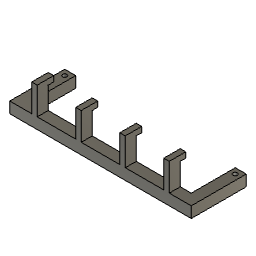
keys holder (Autodesk Fusion 360 design; units mm, degrees)
Autodesk Fusion 360 part; units mm, degrees
sketch "Sketch1" plane through (0, 0, 0) normal (0, 0, 1) x (1, 0, 0)
  line L0 (0, 0) -> (165, 0)
  line L1 (165, 0) -> (165, 50)
  line L2 (165, 50) -> (0, 50)
  line L3 (0, 50) -> (0, 0)
  line L4 (0, 50) -> (10, 50)
  line L5 (10, 50) -> (10, 0)
  line L6 (10, 0) -> (0, 0)
  line L7 (0, 0) -> (0, 50)
  line L8 (165, 50) -> (155, 50)
  line L9 (155, 50) -> (155, 0)
  line L10 (155, 0) -> (165, 0)
  line L11 (165, 0) -> (165, 50)
  line L12 (0, 10) -> (165, 10)
  line L13 (165, 10) -> (165, 0)
  line L14 (165, 0) -> (0, 0)
  line L15 (0, 0) -> (0, 10)
  dimension "d1" = 165
  dimension "d2" = 50
  dimension "d3" = 10
  dimension "d4" = 10
  dimension "d5" = 50
  constraint horizontal L0
  constraint vertical L1
  constraint horizontal L2
  constraint vertical L3
  constraint coincident L0.start L3.end
  constraint horizontal L4
  constraint vertical L5
  constraint horizontal L6
  constraint vertical L7
  constraint horizontal L8
  constraint vertical L9
  constraint horizontal L10
  constraint vertical L11
  constraint horizontal L12
  constraint vertical L13
  constraint horizontal L14
  constraint vertical L15
  constraint coincident L7 L12.start
  measures "d1" distance of L0.start L0.end
  measures "d2" distance of L0.start L2.end
  measures "d3" distance of L2.end L4.end
  measures "d4" distance of L1.end L8.end
  measures "d5" distance of L1.end L0.end
extrude "Extrude1" add sketch "Sketch1" along normal blind 10 contours L0 L3 L5 L6 L7 L12 L14 L15 | L0 L5 L9 L12 L14 | L2 L3 L4 L5 L7 L12 | L0 L1 L9 L10 L11 L12 L13 L14 | L1 L2 L8 L9 L11 L12
sketch "Sketch2" plane through (0, 0, 10) normal (0, 0, 1) x (-1, 0, 0)
  line L0 (-165, 0) -> (-165, -50)
  line L1 (-165, -50) -> (-155, -50)
  line L2 (-155, -50) -> (-155, -10)
  line L3 (-155, -10) -> (-10, -10)
  line L4 (-10, -10) -> (-10, -50)
  line L5 (-10, -50) -> (0, -50)
  line L6 (0, -50) -> (0, 0)
  line L7 (0, 0) -> (-165, 0)
  circle A0 centre (-5, -45) radius 2
  circle A1 centre (-160, -45) radius 2
  dimension "d8" = 4
  dimension "d9" = 4
  measures "d8" diameter of A0
  measures "d9" diameter of A1
extrude "Extrude2" cut sketch "Sketch2" against normal blind 10 contours A0 | A1
sketch "Sketch3" plane through (0, 0, 10) normal (0, 0, 1) x (-1, 0, 0)
  circle A0 centre (-160, -45) radius 2
  circle A1 centre (-5, -45) radius 2
  line L0 (-165, 0) -> (-165, -50)
  line L1 (-165, -50) -> (-155, -50)
  line L2 (-155, -50) -> (-155, -10)
  line L3 (-155, -10) -> (-10, -10)
  line L4 (-10, -10) -> (-10, -50)
  line L5 (-10, -50) -> (0, -50)
  line L6 (0, -50) -> (0, 0)
  line L7 (0, 0) -> (-165, 0)
  line L8 (0, 0) -> (-20, 0)
  line L9 (-20, 0) -> (-25, 0)
  line L10 (-25, 0) -> (-25, -10)
  line L11 (-25, -10) -> (-20, -10)
  line L12 (-20, -10) -> (-20, 0)
  line L13 (-25, 0) -> (-60, 0)
  line L14 (-60, 0) -> (-65, 0)
  line L15 (-65, 0) -> (-65, -10)
  line L16 (-65, -10) -> (-60, -10)
  line L17 (-60, -10) -> (-60, 0)
  line L18 (-65, 0) -> (-100, 0)
  line L19 (-100, 0) -> (-105, 0)
  line L20 (-105, 0) -> (-105, -10)
  line L21 (-105, -10) -> (-100, -10)
  line L22 (-100, -10) -> (-100, 0)
  line L23 (-105, 0) -> (-140, 0)
  line L24 (-140, 0) -> (-145, 0)
  line L25 (-145, 0) -> (-145, -10)
  line L26 (-145, -10) -> (-140, -10)
  line L27 (-140, -10) -> (-140, 0)
  dimension "d12" = 20
  dimension "d13" = 5
  dimension "d14" = 10
  dimension "d15" = 35
  dimension "d16" = 35
  dimension "d17" = 35
  constraint coincident L6.end L7.start
  constraint perpendicular L6 L8
  constraint horizontal L9
  constraint vertical L10
  constraint horizontal L11
  constraint vertical L12
  constraint perpendicular L10 L13
  constraint horizontal L14
  constraint vertical L15
  constraint horizontal L16
  constraint vertical L17
  constraint coincident L3 L15.end
  constraint perpendicular L15 L18
  constraint horizontal L19
  constraint vertical L20
  constraint horizontal L21
  constraint vertical L22
  constraint coincident L3 L20.end
  constraint perpendicular L20 L23
  constraint horizontal L24
  constraint vertical L25
  constraint horizontal L26
  constraint vertical L27
  constraint coincident L3 L25.end
  measures "d12" distance of L6.end L8.end
  measures "d13" distance of L8.end L9.end
  measures "d14" distance of L8.end L11.end
  measures "d15" distance of L9.end L13.end
  measures "d16" distance of L14.end L18.end
  measures "d17" distance of L19.end L23.end
extrude "Extrude3" add sketch "Sketch3" along normal blind 25 contours L3 L7 L24 L25 L26 L27 | L3 L7 L19 L20 L21 L22 | L3 L7 L14 L15 L16 L17 | L3 L7 L9 L10 L11 L12
sketch "Sketch4" plane through (0, 10, 0) normal (0, 1, 0) x (-1, 0, 0)
  line L0 (-155, 0) -> (-10, 0)
  line L1 (-10, 0) -> (-10, 10)
  line L2 (-10, 10) -> (-20, 10)
  line L3 (-20, 10) -> (-20, 35)
  line L4 (-20, 35) -> (-25, 35)
  line L5 (-25, 35) -> (-25, 10)
  line L6 (-25, 10) -> (-60, 10)
  line L7 (-60, 10) -> (-60, 35)
  line L8 (-60, 35) -> (-65, 35)
  line L9 (-65, 35) -> (-65, 10)
  line L10 (-65, 10) -> (-100, 10)
  line L11 (-100, 10) -> (-100, 35)
  line L12 (-100, 35) -> (-105, 35)
  line L13 (-105, 35) -> (-105, 10)
  line L14 (-105, 10) -> (-140, 10)
  line L15 (-140, 10) -> (-140, 35)
  line L16 (-140, 35) -> (-145, 35)
  line L17 (-145, 35) -> (-145, 10)
  line L18 (-145, 10) -> (-155, 10)
  line L19 (-155, 10) -> (-155, 0)
  line L20 (-20, 30) -> (-25, 30)
  line L21 (-25, 30) -> (-25, 35)
  line L22 (-25, 35) -> (-20, 35)
  line L23 (-20, 35) -> (-20, 30)
  line L24 (-60, 30) -> (-65, 30)
  line L25 (-65, 30) -> (-65, 35)
  line L26 (-65, 35) -> (-60, 35)
  line L27 (-60, 35) -> (-60, 30)
  line L28 (-100, 30) -> (-105, 30)
  line L29 (-105, 30) -> (-105, 35)
  line L30 (-105, 35) -> (-100, 35)
  line L31 (-100, 35) -> (-100, 30)
  line L32 (-140, 30) -> (-145, 30)
  line L33 (-145, 30) -> (-145, 35)
  line L34 (-145, 35) -> (-140, 35)
  line L35 (-140, 35) -> (-140, 30)
  constraint horizontal L20
  constraint vertical L21
  constraint horizontal L22
  constraint vertical L23
  constraint coincident L4.end L5.start
  constraint coincident L3 L20.start
  constraint horizontal L24
  constraint vertical L25
  constraint horizontal L26
  constraint vertical L27
  constraint coincident L8.end L9.start
  constraint coincident L7 L24.start
  constraint horizontal L28
  constraint vertical L29
  constraint horizontal L30
  constraint vertical L31
  constraint coincident L12.end L13.start
  constraint coincident L11 L28.start
  constraint horizontal L32
  constraint vertical L33
  constraint horizontal L34
  constraint vertical L35
  constraint coincident L16.end L17.start
  constraint coincident L15 L32.start
extrude "Extrude4" add sketch "Sketch4" along normal blind 5 contours L15 L16 L17 L32 L33 L34 L35 | L3 L4 L5 L20 L21 L22 L23 | L11 L12 L13 L28 L29 L30 L31 | L7 L8 L9 L24 L25 L26 L27
